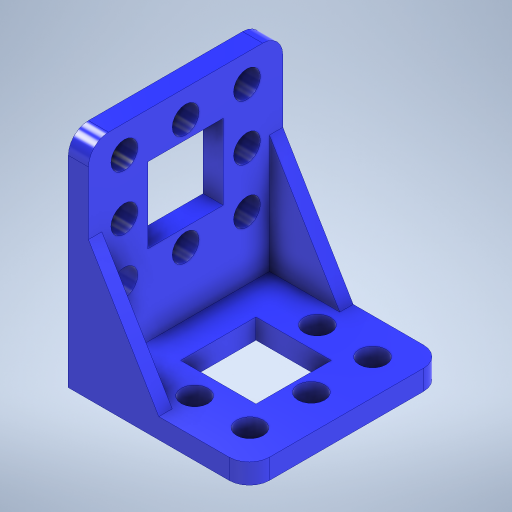
# Autodesk Inventor part: SoporteUnion
Saved by Autodesk Inventor 2023.1 (Build 271208000, 208)
## iProperties
Created: 2023-05-03
Part Number: SoporteUnion
Material: Plastic, Opaque Black
Document SubType Name: Modeling
Designer: felip
Density: 0.952 g/cm^3
Appearance: Blue - Wall Paint - Glossy
Author: felip
Autodesk Inventor part; units mm, degrees
ref_plane "YZ Plane" through (0, 0, 0) normal (1, 0, 0) x (0, 1, 0)
ref_plane "XZ Plane" through (0, 0, 0) normal (0, 1, 0) x (-1, 0, 0)
ref_plane "XY Plane" through (0, 0, 0) normal (0, 0, 1) x (1, 0, 0)
sketch "Sketch1" plane through (0, 0, 0) normal (0, 1, 0) x (-1, 0, 0)
  line L0 (13.5, 14.5) -> (-13.5, 14.5)
  line L1 (-13.5, 14.5) -> (-13.5, -14.5)
  line L2 (-13.5, -14.5) -> (13.5, -14.5)
  line L3 (13.5, -14.5) -> (13.5, 14.5)
  line L4 (5.625, 5.625) -> (-5.625, 5.625)
  line L5 (-5.625, 5.625) -> (-5.625, -5.625)
  line L6 (-5.625, -5.625) -> (5.625, -5.625)
  line L7 (5.625, -5.625) -> (5.625, 5.625)
  circle A0 centre (-8.25, 0) radius 2
  circle A1 centre (-8.25, -9.15) radius 2
  line L8 (-8.25, 0) -> (-4.1919, 0) construction
  circle A2 centre (-8.25, 9.15) radius 2
  line L9 (-4.125, 12.0498) -> (-4.125, -8.6633) construction
  circle A3 centre (0, -9.15) radius 2
  circle A4 centre (0, 9.15) radius 2
  point P0 (0, 0)
  point P1 (-4.125, 1.6932)
  dimension "d0" = 29
  dimension "d1" = 27
  dimension "d2" = 13.5
  dimension "d3" = 14.5
  dimension "d4" = 11.25
  dimension "d5" = 11.25
  dimension "d6" = 5.625
  dimension "d7" = 5.625
  dimension "d8" = 4
  dimension "d9" = 5.25
  dimension "d10" = 4
  dimension "d12" = 5.35
  dimension "d13" = 4.125
  dimension "d23" = 2.625
  dimension "d40" = 9.15
  dimension "d41" = 8.25
  constraints: 20 end point, 5 centre point, 4 parallel, 3 perpendicular, 3 symmetric about line, 2 horizontal, 1 midpoint, 1 vertical, 3 other
  measures "d0" distance of L0.end L1.end
  measures "d1" distance of L0.start L0.end
  measures "d2" distance from line of point (0, 0) L3
  measures "d3" distance from line of point (0, 0) L0
  measures "d4" distance of L6.end L4.start
  measures "d5" distance of L4.start L4.end
  measures "d6" distance from line of point (0, 0) L7
  measures "d7" distance from line of point (0, 0) L4
  measures "d8" diameter of A0
  measures "d9" distance from line of L1 L8.start
  measures "d10" diameter of A1
  measures "d12" distance from line of L2 A1.centre
  measures "d13" horizontal distance of point (-4.125, 1.693) point (0, 0)
  measures "d23" distance from line of L8.start L5
  measures "d40" distance of L8.start A1.centre
  measures "d41" distance of A3.centre A1.centre
extrude "Extrusion1" add sketch "Sketch1" along normal blind 3
fillet "Fillet1" radius 3 2 edges at (13.5, 1.5, 14.5) (13.5, 1.5, -14.5)
sketch "Sketch2" plane through (-13.5, 0, -14.5) normal (-1, 0, 0) x (0, 0, 1)
  line L0 (0, 0) -> (0, 3) projected
  line L1 (0, 0) -> (29, 0)
  line L2 (29, 0) -> (29, 33)
  line L3 (29, 33) -> (0, 33)
  line L4 (0, 33) -> (0, 0)
  line L5 (0, 3) -> (29, 3) projected
  line L6 (8.875, 26.25) -> (20.125, 26.25)
  line L7 (20.125, 26.25) -> (20.125, 15)
  line L8 (20.125, 15) -> (8.875, 15)
  line L9 (8.875, 15) -> (8.875, 26.25)
  circle A0 centre (14.5, 12.375) radius 2
  circle A1 centre (23.65, 12.375) radius 2
  line L10 (3.2403, 20.625) -> (27.5408, 20.625) construction
  line L11 (14.5, 12.375) -> (14.5, 30.5106) construction
  circle A2 centre (5.35, 12.375) radius 2
  circle A3 centre (14.5, 28.875) radius 2
  circle A4 centre (23.65, 28.875) radius 2
  circle A5 centre (5.35, 28.875) radius 2
  line L12 (2.8915, 16.5) -> (25.3317, 16.5) construction
  circle A6 centre (23.65, 28.875) radius 2
  circle A7 centre (5.35, 28.875) radius 2
  circle A8 centre (23.65, 20.625) radius 2
  circle A9 centre (5.35, 20.625) radius 2
  point P0 (14.5, 0)
  dimension "d17" = 29
  dimension "d18" = 33
  dimension "d19" = 11.25
  dimension "d20" = 11.25
  dimension "d21" = 12
  dimension "d22" = 8.875
  dimension "d24" = 4
  dimension "d25" = 2.625
  dimension "d26" = 4
  dimension "d27" = 5.35
  dimension "d28" = 0
  dimension "d29" = 5.625
  dimension "d30" = 5.625
  dimension "d31" = 8.25
  dimension "d32" = 4.125
  constraints: 22 end point, 10 centre point, 8 symmetric about line, 4 horizontal, 4 parallel, 2 perpendicular, 1 vertical, 8 other
  measures "d17" distance of L3.end L2.end
  measures "d18" distance of L2.end L1.end
  measures "d19" distance of L7.end L8.end
  measures "d20" distance of L6.end L7.end
  measures "d21" distance between parallel lines of L5 L8
  measures "d22" distance between parallel lines of L4 L9
  measures "d24" diameter of A0
  measures "d25" distance from line of L11.start L8
  measures "d26" diameter of A1
  measures "d27" distance from line of L2 A1.centre
  measures "d28" vertical distance of L11.start A1.centre
  measures "d29" distance between parallel lines of L10 L6
  measures "d30" distance between parallel lines of L11 L9
  measures "d31" distance from line of L11.start L10
  measures "d32" distance between parallel lines of L12 L10
extrude "Extrusion2" add sketch "Sketch2" against normal blind 3 contours L4 L3 L2 L5
fillet "Fillet2" radius 3 2 edges at (-12, 33, 14.5) (-12, 33, -14.5)
sketch "Sketch3" plane through (-13.5, 0, 14.5) normal (0, 0, 1) x (1, 0, 0)
  line L0 (0, 18.625) -> (0, 22.625) projected
  line L1 (11.5, 3) -> (15.5, 3) projected
  line L2 (3, 22.625) -> (3, 18.625) projected
  line L3 (3, 22.625) -> (3, 18.625) projected
  line L4 (3, 20.625) -> (13.5, 3)
  line L5 (19.125, 3) -> (7.875, 3) projected
  line L6 (3, 30) -> (3, 3) projected
  line L7 (3, 3) -> (24, 3) projected
  point P0 (13.5, 0)
  constraints: 2 end point, 2 midpoint
extrude "Extrusion3" add sketch "Sketch3" against normal blind 2
sketch "Sketch4" plane through (10.5, 0, -14.5) normal (0, 0, -1) x (-1, 0, 0)
  line L0 (10.5, 3) -> (21, 20.625) projected
  line L1 (21, 20.625) -> (21, 3) projected
  line L2 (21, 3) -> (10.5, 3) projected
  point P0 (10.5, 0)
extrude "Extrusion4" add sketch "Sketch4" against normal blind 2
equation "\"d2\" = 0.5 * d1"
equation "\"d3\" = 0.5 * d0"
equation "\"d5\" = d4"
equation "\"d6\" = 0.5 * d5"
equation "\"d7\" = 0.5 * d4"
equation "\"d13\" = -0.5 * d9 + 0.5 * d2"
equation "\"d20\" = d19"
equation "\"d22\" = 0.5 * d17 - 0.5 * d19"
equation "\"d26\" = d24"
equation "\"d29\" = 0.5 * d20"
equation "\"d30\" = d29"
equation "\"d32\" = 0.5 * d31"
body "Solid1"
